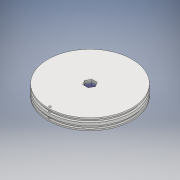
# Autodesk Inventor part: PulleyWithHole
Saved by Autodesk Inventor 2017 (Build 210142000, 142)
## iProperties
Created: 2017-02-11
Part Number: PulleyWithHole
Material: ABS Plastic
Document SubType Name: Modeling
Designer: aribu
Density: 1.06 g/cm^3
Appearance: Smooth - White
Mass: 23.3866 g
Surface Area: 86.2287 cm^2
Volume: 22.0629 cm^3
Author: aribu
Autodesk Inventor part; units mm, degrees
ref_plane "YZ Plane" through (0, 0, 0) normal (1, 0, 0) x (0, 1, 0)
ref_plane "XZ Plane" through (0, 0, 0) normal (0, 1, 0) x (-1, 0, 0)
ref_plane "XY Plane" through (0, 0, 0) normal (0, 0, 1) x (1, 0, 0)
sketch "Sketch3" plane through (0, 0, 0) normal (0, 0, 1) x (1, 0, 0)
  circle A0 centre (0, 0) radius 4.45
  dimension "d11" = 8.9
  constraints: 1 centre point, 1 coincident
  measures "d11" diameter of A0
extrude "Extrusion3" add sketch "Sketch3" along normal blind 6
sketch "Sketch4" plane through (0, 0, 6) normal (0, 0, 1) x (1, 0, 0)
  circle A0 centre (0, 0) radius 30
  dimension "d14" = 60
  constraints: 1 centre point, 1 coincident
  measures "d14" diameter of A0
extrude "Extrusion4" add sketch "Sketch4" along normal blind 8
ref_plane "Work Plane2" through (0, 0, 8) normal (0, 0, 1) x (1, 0, 0)
ref_plane "Work Plane1" through (0, 0, 10) normal (0, 0, 1) x (1, 0, 0)
sketch "Sketch5" plane through (0, 0, 8) normal (0, 0, 1) x (1, 0, 0)
  arc A0 (0.5639, -28.4944) -> (-0.5169, -28.4953) centre (0, 0) ccw
  circle A1 centre (0, 0) radius 30
  line L0 (0.5639, -28.4944) -> (0.5639, -23.859)
  line L1 (0.5639, -23.859) -> (-0.5169, -23.859)
  line L2 (-0.5169, -23.859) -> (-0.5169, -28.4953)
  dimension "d17" = 57
  dimension "d18" = 60
  constraints: 6 end point, 2 centre point, 2 coincident, 2 point on circle, 1 parallel
  measures "d17" diameter of A0
  measures "d18" diameter of A1
extrude "Extrusion5" cut sketch "Sketch5" along normal mid plane 2
mirror "Mirror1" about plane through (0, 0, 10) normal (0, 0, 1) of "Extrusion5"
sketch "Sketch9" plane through (0, 0, 0) normal (0, 0, -1) x (-1, 0, 0)
  circle A0 centre (0, 0) radius 4.45 projected
  circle A1 centre (0, 0) radius 4.45
  dimension "d40" = 8.9
  constraints: 1 centre point, 1 coincident
  measures "d40" diameter of A1
extrude "Extrusion9" cut sketch "Sketch9" against normal blind 6
sketch "Sketch10" plane through (0, 0, 14) normal (0, 0, 1) x (1, 0, 0)
  circle A0 centre (0, -28.6156) radius 0.75
  point P0 (0, 0)
  dimension "d43" = 1.5
  constraints: 1 centre point
  measures "d43" diameter of A0
extrude "Extrusion10" cut sketch "Sketch10" against normal blind 10
sketch "Sketch11" plane through (0, 0, 14) normal (0, 0, 1) x (1, 0, 0)
  line L0 (1.9038, -3.3009) -> (-1.9068, -3.2991)
  line L1 (-1.9068, -3.2991) -> (-3.8105, 0.0017)
  line L2 (-3.8105, 0.0017) -> (-1.9038, 3.3009)
  line L3 (-1.9038, 3.3009) -> (1.9068, 3.2991)
  line L4 (1.9068, 3.2991) -> (3.8105, -0.0017)
  line L5 (3.8105, -0.0017) -> (1.9038, -3.3009)
  point P0 (0, 0)
  point P1 (0, 0)
  dimension "d46" = 6.6
  constraints: 12 end point, 1 coincident, 13 other
  measures "d46" distance between parallel lines of L0 L3
extrude "Extrusion11" cut sketch "Sketch11" against normal blind 10
ref_plane "Work Plane3" through (0, 0, 10) normal (0, 0, 1) x (1, 0, 0)
ref_plane "Work Plane4" through (0, 0, 12) normal (0, 0, 1) x (1, 0, 0)
body "Solid2"
